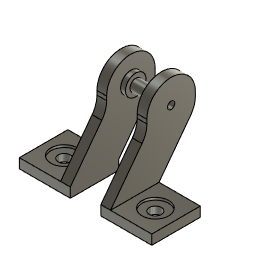
gear (Autodesk Fusion 360 design; units mm, degrees)
Autodesk Fusion 360 part; units mm, degrees
sketch "Sketch1" plane through (0, 0, 0) normal (0, 0, 1) x (1, 0, 0) in component "Linker Teil"
  line L0 (0, 0) -> (21, 0)
  line L1 (21, 0) -> (21, 20)
  line L2 (21, 20) -> (0, 20)
  line L3 (0, 20) -> (0, 0)
  dimension "d1" = 20
  dimension "d2" = 21
  constraint horizontal L0
  constraint vertical L1
  constraint horizontal L2
  constraint vertical L3
  constraint coincident L0.start L3.end
  measures "d1" distance of L0.start L2.end
  measures "d2" distance of L0.start L0.end
extrude "Extrude1" add sketch "Sketch1" along normal blind 4 makes body 1 in component "Linker Teil"
sketch "Schraubenkopf" plane through (0, 0, 4) normal (0, 0, 1) x (-1, 0, 0) in component "Linker Teil"
  line L0 (0, -20) -> (0, 0)
  line L1 (0, 0) -> (-21, 0)
  line L2 (-21, 0) -> (-21, -20)
  line L3 (-21, -20) -> (0, -20)
  circle A0 centre (-8.5, -10) radius 5.5
  dimension "d10" = 11
  dimension "d11" = 8.5
  dimension "d12" = 10
  measures "d10" diameter of A0
  measures "d11" distance of L0 A0.centre
  measures "d12" distance of L3 A0.centre
extrude "Extrude2" cut sketch "Schraubenkopf" against normal blind 1 contours A0 bodies 1 in component "Linker Teil"
sketch "Schraubenbohrung" plane through (0, 0, 3) normal (0, 0, 1) x (-1, 0, 0) in component "Linker Teil"
  circle A0 centre (-8.5, -10) radius 5.5
  circle A1 centre (-8.5, -10) radius 2.5
  dimension "d15" = 5
  constraint concentric A0 A1
  measures "d15" diameter of A1
extrude "Extrude3" cut sketch "Schraubenbohrung" against normal up to surface (3 mm away) contours A1 bodies 1 in component "Linker Teil"
sketch "Sketch4" plane through (21, 0, 0) normal (1, 0, 0) x (0, 1, 0) in component "Linker Teil"
  line L0 (0, 0) -> (20, 0)
  line L1 (20, 0) -> (20, 4)
  line L2 (20, 4) -> (0, 4)
  line L3 (0, 4) -> (0, 0)
  line L4 (20, 4) -> (35, 24)
  line L5 (15, 24) -> (0, 4)
  line L6 (15, 24) -> (35, 24) construction
  line L7 (35, 24) -> (35, 29)
  line L8 (15, 29) -> (15, 24)
  line L9 (35, 29) -> (15, 29) construction
  arc A0 (35, 29) -> (15, 29) centre (25, 29) ccw
  dimension "d18" = 20
  dimension "d19" = 15
  dimension "d22" = 20
  dimension "d23" = 5
  constraint coincident L1.end L2.start
  constraint coincident L2.end L3.start
  constraint horizontal L6
  constraint vertical L7
  constraint vertical L8
  constraint coincident L4.end L6.end
  constraint tangent L8 A0
  constraint tangent L7 A0
  measures "d18" distance of L4.end L5.start
  measures "d19" horizontal distance of L1.end L4.end
  measures "d22" vertical distance of L1.end L4.end
  measures "d23" distance of L4.end L7.end
extrude "Extrude4" add sketch "Sketch4" against normal blind 4 contours L2 L4 L5 L7 L8 A0 bodies 1 in component "Linker Teil"
sketch "Distanzhalter" plane through (21, 0, 0) normal (1, 0, 0) x (0, 1, 0) in component "Linker Teil"
  line L0 (0, 0) -> (20, 0)
  line L1 (20, 0) -> (20, 4)
  line L2 (20, 4) -> (35, 24)
  line L3 (35, 24) -> (35, 29)
  arc A0 (35, 29) -> (15, 29) centre (25, 29) ccw
  line L4 (15, 29) -> (15, 24)
  line L5 (15, 24) -> (0, 4)
  line L6 (0, 4) -> (0, 0)
  circle A1 centre (25, 29) radius 4.25
  dimension "d27" = 8.5
  constraint concentric A0 A1
  measures "d27" diameter of A1
extrude "Extrude5" add sketch "Distanzhalter" along normal blind 2 contours A1 bodies 1 in component "Linker Teil"
sketch "Zahnradhalterung" plane through (23, 0, 0) normal (1, 0, 0) x (0, 1, 0) in component "Linker Teil"
  circle A0 centre (25, 29) radius 4.25
  circle A1 centre (25, 29) radius 2.4
  dimension "d30" = 4.8
  constraint concentric A0 A1
  measures "d30" diameter of A1
extrude "Extrude6" add sketch "Zahnradhalterung" along normal blind 11.1 contours A1 bodies 1 in component "Linker Teil"
sketch "Sketch8" plane through (34.1, 0, 0) normal (1, 0, 0) x (0, 1, 0) in component "Linker Teil"
  circle A0 centre (25, 29) radius 2.4
  circle A1 centre (25, 29) radius 1.5
  dimension "d33" = 3
  constraint concentric A0 A1
  measures "d33" diameter of A1
extrude "Extrude7" cut sketch "Sketch8" against normal up to surface (17.1 mm away) contours A1 bodies 1 in component "Linker Teil"
sketch "Distanzhalter (2)" plane through (34.1, 0, 0) normal (1, 0, 0) x (0, 1, 0) in component "Rechter Teil"
  circle A0 through (29.2245, 29, -2.5) (22.8878, 32.6585, -2.5) (22.8878, 25.3415, -2.5)
extrude "Extrude1'" add sketch "Distanzhalter (2)" along normal blind 2 separate body contours A0 in plane through (31.6, 0, 0) normal (1, 0, 0) makes body 2 in component "Rechter Teil"
sketch "Sketch2" plane through (33.6, 0, 0) normal (1, 0, 0) x (0, 1, 0) in component "Rechter Teil"
  line L0 (15, 29) -> (29.2245, 29) construction
  line L1 (35, 29) -> (35, 24)
  line L2 (35, 24) -> (15, 24) construction
  line L3 (15, 24) -> (15, 29)
  line L4 (15, 24) -> (0, 4)
  line L5 (0, 4) -> (20, 4)
  line L6 (20, 4) -> (35, 24)
  arc A0 (35, 29) -> (15, 29) centre (25, 29) ccw
  dimension "d38" = 20
  dimension "d39" = 5
  dimension "d40" = 20
  dimension "d41" = 15
  constraint horizontal L0
  constraint vertical L1
  constraint horizontal L2
  constraint vertical L3
  constraint tangent L3 A0
  constraint tangent L1 A0
  constraint perpendicular L3 L5
  constraint parallel L4 L6
  measures "d38" diameter of A0
  measures "d39" distance of L0.start L2.end
  measures "d40" vertical distance of L2.end L4.end
  measures "d41" horizontal distance of L2.end L4.end
extrude "Extrude2'" add sketch "Sketch2" along normal blind 4 bodies 2 in component "Rechter Teil"
sketch "Sketch3" plane through (0, 0, 4) normal (0, 0, -1) x (1, 0, 0) in component "Rechter Teil"
  line L0 (33.6, 0) -> (33.6, -20)
  line L1 (33.6, -20) -> (37.6, -20)
  line L2 (37.6, -20) -> (37.6, 0) construction
  line L3 (37.6, 0) -> (33.6, 0)
  line L4 (33.6, 0) -> (54.6, 0)
  line L5 (54.6, 0) -> (54.6, -20)
  line L6 (33.6, -20) -> (33.6, 0)
  line L7 (54.6, -20) -> (33.6, -20)
  dimension "d44" = 21
  constraint horizontal L4
  constraint vertical L5
  constraint vertical L6
  constraint coincident L0.start L3.end
  constraint coincident L0.end L1.start
  constraint perpendicular L0 L7
  measures "d44" distance of L0.start L4.end
extrude "Extrude3'" add sketch "Sketch3" along normal blind 4 bodies 2 in component "Rechter Teil"
sketch "Sketch4 (2)" plane through (31.6, 0, 0) normal (-1, 0, 0) x (0, -1, 0) in component "Rechter Teil"
  circle A0 centre (-25, 29) radius 4.2245
  circle A1 centre (-25, 29) radius 2.5
  dimension "d47" = 5
  constraint concentric A0 A1
  measures "d47" diameter of A1
extrude "Extrude4'" cut sketch "Sketch4 (2)" against normal blind 3 contours A1 bodies 2 in component "Rechter Teil"
sketch "Bohrloch" plane through (34.6, 0, 0) normal (-1, 0, 0) x (0, -1, 0) in component "Rechter Teil"
  circle A0 centre (-25, 29) radius 2.5
  circle A1 centre (-25, 29) radius 1.5
  dimension "d50" = 3
  constraint concentric A0 A1
  measures "d50" diameter of A1
extrude "Extrude5'" cut sketch "Bohrloch" against normal up to surface (3 mm away) contours A1 bodies 2 in component "Rechter Teil"
sketch "Sketch6" plane through (0, 0, 4) normal (0, 0, 1) x (-1, 0, 0) in component "Rechter Teil"
  line L0 (-37.6, -20) -> (-37.6, 0)
  line L1 (-37.6, 0) -> (-54.6, 0)
  line L2 (-54.6, 0) -> (-54.6, -20)
  line L3 (-54.6, -20) -> (-37.6, -20)
  circle A0 centre (-46.1, -10) radius 5.5
  dimension "d53" = 11
  dimension "d54" = 10
  dimension "d55" = 8.5
  measures "d53" diameter of A0
  measures "d54" distance of L3 A0.centre
  measures "d55" distance of L2 A0.centre
extrude "Extrude6'" cut sketch "Sketch6" against normal blind 1 contours A0 bodies 2 in component "Rechter Teil"
sketch "Sketch7" plane through (0, 0, 3) normal (0, 0, 1) x (-1, 0, 0) in component "Rechter Teil"
  circle A0 centre (-46.1, -10) radius 5.5
  circle A1 centre (-46.1, -10) radius 2.5
  dimension "d58" = 5
  constraint concentric A0 A1
  measures "d58" diameter of A1
extrude "Extrude7'" cut sketch "Sketch7" against normal up to surface (3 mm away) contours A1 bodies 2 in component "Rechter Teil"
fillet "Fillet1" radius 10 2 edges at (35.6, 35, 24) (35.6, 15, 24) on bodies 2 in component "Rechter Teil"
fillet "Fillet1'" radius 10 2 edges at (19, 15, 24) (19, 35, 24) on bodies 1 in component "Linker Teil"
component "Linker Teil" placed x (1, 0, 0) y (0, 1, 0) z (0, 0, 1) at (0, 0, 0)
component "Rechter Teil" placed x (1, 0, 0) y (0, 1, 0) z (0, 0, 1) at (0, 0, 0)
